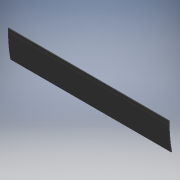
# Autodesk Inventor part: base
Saved by Autodesk Inventor 2018.1 (Build 221171000, 171)
## iProperties
Created: 2017-10-18
Part Number: base
Material: CFRP
Document SubType Name: Modeling
Designer: kuwano
Density: 1.43 g/cm^3
Appearance: カーボンファイバー
Mass: 2365.86 g
Surface Area: 6778.95 cm^2
Volume: 1654.45 cm^3
Author: kuwano
Autodesk Inventor part; units mm, degrees
ref_plane "YZ Plane" through (0, 0, 0) normal (1, 0, 0) x (0, 1, 0)
ref_plane "XZ Plane" through (0, 0, 0) normal (0, 1, 0) x (-1, 0, 0)
ref_plane "XY Plane" through (0, 0, 0) normal (0, 0, 1) x (1, 0, 0)
sketch "スケッチ2" plane through (0, 0, 0) normal (1, 0, 0) x (0, 1, 0)
  arc A0 (-5, 100) -> (15.0899, -110.9438) centre (1112.5, 100) ccw
  arc A1 (0, 100) -> (20, -110) centre (1112.5, 100) ccw
  line L0 (0, 100) -> (-5, 100)
  line L1 (20, -110) -> (15.0899, -110.9438)
  line L2 (0, -153.7053) -> (0, 142.2842) projected
  line L3 (-234.5134, 0) -> (1337.0022, 0) projected
  point P0 (0, 0)
  dimension "d5" = 5
  dimension "d6" = 100
  dimension "d9" = 20
  dimension "d10" = 110
  constraints: 4 end point, 4 line through centre, 4 point on circle, 2 centre point, 1 concentric, 1 point on line, 1 tangent
  measures "d5" radial gap between concentric circles of A0 A1
  measures "d6" distance from line of L3 L0.start
  measures "d9" distance from line of L2 L1.start
  measures "d10" distance from line of L3 L1.start
extrude "押し出し2" add sketch "スケッチ2" along normal mid plane 1370
sketch "スケッチ3" plane through (-685, -5, 100) normal (0, 0, 1) x (1, 0, 0)
  line L0 (0, 0) -> (1370, 0) projected
  line L1 (1370, 5) -> (1370, 0) projected
  line L2 (0, 0) -> (1370, 0)
  line L3 (1370, 0) -> (1370, 5)
  line L4 (1370, 5) -> (0, 5)
  line L5 (0, 5) -> (0, 0)
  point P0 (685, 5)
  constraints: 8 end point, 2 parallel, 1 horizontal, 1 perpendicular
extrude "押し出し3" add sketch "スケッチ3" along normal blind 30
